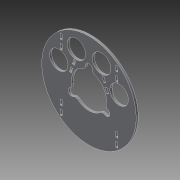
# Autodesk Inventor part: М_П_Основание верхнее
Saved by Autodesk Inventor 2022 (Build 260153000, 153)
## iProperties
Created: 2025-01-25
Part Number: М_П_Основание верхнее
Material: Типовые
Document SubType Name: Modeling
Designer: Ivan
Density: 1 g/cm^3
Appearance: По умолчанию
Author: Ivan
Autodesk Inventor part; units mm, degrees
ref_plane "YZ Plane" through (0, 0, 0) normal (1, 0, 0) x (0, 1, 0)
ref_plane "XZ Plane" through (0, 0, 0) normal (0, 1, 0) x (-1, 0, 0)
ref_plane "XY Plane" through (0, 0, 0) normal (0, 0, 1) x (1, 0, 0)
ref_plane "РабПлоскость1" through (48.3327, 32.65, 41) normal (0, 0, 1) x (-0.3420201, 0.9396926, 0)
sketch "Эскиз1" plane through (48.3327, 32.65, 41) normal (0, 0, 1) x (-0.3420201, 0.9396926, 0)
  circle A0 centre (-58.1978, 19.6246) radius 1.6 projected
  circle A1 centre (-24.135, 113.2113) radius 1.6 projected
  circle A2 centre (39.8821, 36.9187) radius 1.6 projected
  circle A3 centre (-14.1502, 56.5848) radius 135 projected
  line L0 (29.5378, -47.49) -> (15.4424, -42.3597) projected
  line L1 (15.4424, -42.3597) -> (17.4946, -36.7216) projected
  line L2 (17.4946, -36.7216) -> (31.59, -41.8519) projected
  line L3 (31.59, -41.8519) -> (29.5378, -47.49) projected
  line L4 (-69.2873, 158.4418) -> (-83.3827, 163.5721) projected
  line L5 (-83.3827, 163.5721) -> (-81.3306, 169.2102) projected
  line L6 (-81.3306, 169.2102) -> (-67.2352, 164.0799) projected
  line L7 (-67.2352, 164.0799) -> (-69.2873, 158.4418) projected
  line L8 (42.6503, 86.706) -> (54.141, 77.0642) projected
  line L9 (54.141, 77.0642) -> (50.2843, 72.4679) projected
  line L10 (50.2843, 72.4679) -> (38.7936, 82.1098) projected
  line L11 (38.7936, 82.1098) -> (42.6503, 86.706) projected
  line L12 (84.1627, 102.5905) -> (70.0673, 107.7208) projected
  line L13 (70.0673, 107.7208) -> (72.1194, 113.359) projected
  line L14 (72.1194, 113.359) -> (86.2148, 108.2287) projected
  line L15 (86.2148, 108.2287) -> (84.1627, 102.5905) projected
  line L16 (-112.4631, 10.5792) -> (-98.3677, 5.4489) projected
  line L17 (-98.3677, 5.4489) -> (-100.4198, -0.1893) projected
  line L18 (-100.4198, -0.1893) -> (-114.5152, 4.941) projected
  line L19 (-114.5152, 4.941) -> (-112.4631, 10.5792) projected
  line L20 (10, 3) -> (25, 3) projected
  line L21 (25, 3) -> (25, -3) projected
  line L22 (25, -3) -> (10, -3) projected
  line L23 (10, -3) -> (10, 3) projected
  line L24 (0, 3) -> (0, -3) projected
  line L25 (0, -3) -> (-15, -3) projected
  line L26 (-15, -3) -> (-15, 3) projected
  line L27 (-15, 3) -> (0, 3) projected
  line L28 (-121.86, 13.9994) -> (-123.9122, 8.3612) projected
  line L29 (-123.9122, 8.3612) -> (-138.0076, 13.4915) projected
  line L30 (-138.0076, 13.4915) -> (-135.9554, 19.1297) projected
  line L31 (-135.9554, 19.1297) -> (-121.86, 13.9994) projected
  line L32 (93.5596, 99.1703) -> (95.6117, 104.8085) projected
  line L33 (95.6117, 104.8085) -> (109.7071, 99.6782) projected
  line L34 (109.7071, 99.6782) -> (107.655, 94.04) projected
  line L35 (107.655, 94.04) -> (93.5596, 99.1703) projected
  circle A4 centre (-14.1502, 56.5848) radius 50 projected
  line L36 (34.9899, 93.1339) -> (31.1332, 88.5376) projected
  line L37 (31.1332, 88.5376) -> (19.6425, 98.1795) projected
  line L38 (19.6425, 98.1795) -> (23.4992, 102.7757) projected
  line L39 (23.4992, 102.7757) -> (34.9899, 93.1339) projected
  line L40 (-59.8904, 155.0216) -> (-57.8383, 160.6597) projected
  line L41 (-57.8383, 160.6597) -> (-43.7429, 155.5294) projected
  line L42 (-43.7429, 155.5294) -> (-45.795, 149.8913) projected
  line L43 (-45.795, 149.8913) -> (-59.8904, 155.0216) projected
  line L44 (38.9348, -50.9102) -> (40.9869, -45.2721) projected
  line L45 (40.9869, -45.2721) -> (55.0823, -50.4024) projected
  line L46 (55.0823, -50.4024) -> (53.0301, -56.0405) projected
  line L47 (53.0301, -56.0405) -> (38.9348, -50.9102) projected
  circle A5 centre (78.223, 61.4259) radius 24 construction
  circle A6 centre (53.5, -6.5) radius 24 construction
  circle A7 centre (46.5352, 126.3955) radius 24 construction
  circle A8 centre (-12.5359, -35.9011) radius 24 construction
  circle A9 centre (-12.5359, -35.9011) radius 26.5
  circle A10 centre (53.5, -6.5) radius 26.5
  circle A11 centre (78.223, 61.4259) radius 26.5
  circle A12 centre (46.5352, 126.3955) radius 26.5
  point P0 (-14.1502, 56.5848)
  dimension "d2" = 53
  constraints: 4 centre point, 4 coincident, 3 equal radius
  measures "d2" diameter of A9
extrude "Выдавливание1" add sketch "Эскиз1" along normal blind 6
sketch "Эскиз2" plane through (0, 0, 47) normal (0, 0, 1) x (1, 0, 0)
  circle A0 centre (0, 57.5) radius 1.6 projected
  circle A1 centre (0, 57.5) radius 1.6 projected
  circle A2 centre (0, 57.5) radius 10
  point P0 (0, 0)
  dimension "d3" = 20
  constraints: 1 centre point, 1 coincident
  measures "d3" diameter of A2
extrude "Выдавливание2" cut sketch "Эскиз2" against normal through all
fillet "Сопряжение1" radius 10 2 edges at (-6.1562, 49.6196, 44) (6.1562, 49.6196, 44)
pattern_circular "Круговой массив1" count 3 over 360 about axis through (0, 0, 41) along (0, 0, 1) of "Сопряжение1", "Выдавливание2"
